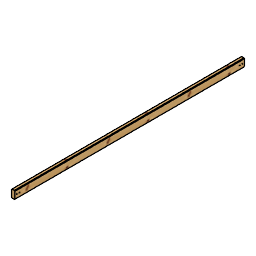
_2x4 board.d99266e9-60ea-4329-bf0e-f758237543eb (Autodesk Fusion 360 design; units mm, degrees)
Autodesk Fusion 360 part; units mm, degrees
sketch "Sketch1" plane through (0, 0, 0) normal (0, 0, 1) x (1, 0, 0)
  line L0 (5, 0) -> (33.1, 0)
  line L1 (38.1, 5) -> (38.1, 83.9)
  line L2 (33.1, 88.9) -> (5, 88.9)
  line L3 (0, 83.9) -> (0, 5)
  arc A0 (38.1, 83.9) -> (33.1, 88.9) centre (33.1, 83.9) ccw
  arc A1 (5, 88.9) -> (0, 83.9) centre (5, 83.9) ccw
  arc A2 (0, 5) -> (5, 0) centre (5, 5) ccw
  arc A3 (33.1, 0) -> (38.1, 5) centre (33.1, 5) ccw
  point P0 (38.1, 0)
  point P1 (0, 88.9)
  dimension "d1" = 38.1
  dimension "d2" = 88.9
  dimension "d3" = 5
  constraint horizontal L0
  constraint vertical L1
  constraint horizontal L2
  constraint vertical L3
  constraint tangent L1 A0
  constraint tangent L2 A0
  constraint coincident P1 L2
  constraint coincident P1 L3
  constraint tangent L2 A1
  constraint tangent L3 A1
  constraint equal A0 A1
  constraint coincident origin L0
  constraint coincident origin L3
  constraint tangent L0 A2
  constraint tangent L3 A2
  constraint equal A0 A2
  constraint coincident P0 L0
  constraint coincident P0 L1
  constraint tangent L0 A3
  constraint tangent L1 A3
  constraint equal A0 A3
  measures "d1" distance of origin P0
  measures "d2" distance of origin P1
  measures "d3" radius of A0
extrude "Extrude1" add sketch "Sketch1" along normal blind 2590.8
sketch "Sketch2" plane through (38.1, 0, 0) normal (1, 0, 0) x (0, 0, -1)
  line L0 (0, 5) -> (0, 83.9)
  line L1 (0, 83.9) -> (-2590.8, 83.9)
  line L2 (-2590.8, 83.9) -> (-2590.8, 5)
  line L3 (-2590.8, 5) -> (0, 5)
  line L4 (0, 44.45) -> (-22.9, 44.45) construction
  circle A0 centre (-22.9, 44.45) radius 5
  line L5 (-22.9, 44.45) -> (-53.289, 44.45) construction
  circle A1 centre (-53.289, 44.45) radius 5
  circle A2 centre (-2537.511, 44.45) radius 5
  circle A3 centre (-2567.9, 44.45) radius 5
  line L6 (-2590.8, 44.45) -> (-2567.9, 44.45) construction
  line L7 (-2567.9, 44.45) -> (-2537.511, 44.45) construction
  dimension "d6" = 22.9
  dimension "d7" = 10
  dimension "d8" = 30.389
  dimension "d9" = 10
  dimension "d10" = 22.9
  dimension "d11" = 10
  dimension "d12" = 30.389
  dimension "d13" = 10
  constraint midpoint L0 L4.start
  constraint perpendicular L0 L4
  constraint coincident L4.end A0.centre
  constraint parallel L4 L5
  constraint coincident L5.end A1.centre
  constraint coincident A3.centre L6.end
  constraint parallel L6 L7
  constraint coincident A2.centre L7.end
  constraint midpoint L2 L6.start
  constraint perpendicular L2 L6
  measures "d6" distance of L4.start L4.end
  measures "d7" diameter of A0
  measures "d8" distance of L4.end L5.end
  measures "d9" diameter of A1
  measures "d10" distance of A3.centre L6.start
  measures "d11" diameter of A3
  measures "d12" distance of A3.centre A2.centre
  measures "d13" diameter of A2
extrude "Extrude2" cut sketch "Sketch2" against normal up to surface (38.1 mm away) contours A0 | A1 | A2 | A3
